Autodesk Inventor part; units mm, degrees
(part 3 of 3)
sketch "スケッチ5" plane through (0, 0, 6) normal (0, 0, 1) x (1, 0, 0)
  line L0 (155.6611, 116.5538) -> (164.0413, 130.0744) projected
  line L1 (164.0413, 130.0744) -> (164.3416, 130.559) projected
  arc A0 (164.3416, 130.559) -> (164.502, 130.8893) centre (161.9481, 131.9254) ccw projected
  arc A1 (164.502, 130.8893) -> (164.8829, 132.1201) centre (157.4972, 133.7312) ccw projected
  arc A2 (164.8829, 132.1201) -> (165.1789, 134.6281) centre (152.1823, 134.8905) ccw projected
  arc A3 (165.1789, 134.6281) -> (163.8683, 135.3286) centre (148.5, 105.0002) ccw projected
  arc A4 (163.8683, 135.3286) -> (161.9475, 133.6891) centre (171.3071, 124.6681) ccw projected
  arc A5 (161.9475, 133.6891) -> (161.1357, 132.6886) centre (167.3903, 128.4432) ccw projected
  arc A6 (161.1357, 132.6886) -> (160.9502, 132.3718) centre (163.4161, 131.1408) ccw projected
  line L2 (160.9502, 132.3718) -> (160.7141, 131.8528) projected
  arc A7 (160.7141, 131.8528) -> (158.8509, 132.6246) centre (148.5, 105.0002) ccw projected
  line L3 (158.8509, 132.6246) -> (159.051, 133.1584) projected
  arc A8 (159.051, 133.1584) -> (159.1439, 133.5137) centre (156.4368, 134.0317) ccw projected
  arc A9 (159.1439, 133.5137) -> (159.2773, 134.7951) centre (151.7192, 134.9344) ccw projected
  arc A10 (159.2773, 134.7951) -> (159.0783, 137.3127) centre (146.2802, 135.0346) ccw projected
  arc A11 (159.0783, 137.3127) -> (157.6563, 137.744) centre (148.5, 105.0002) ccw projected
  arc A12 (157.6563, 137.744) -> (156.0922, 135.7613) centre (167.0319, 128.7396) ccw projected
  arc A13 (156.0922, 135.7613) -> (155.4912, 134.6217) centre (162.4539, 131.678) ccw projected
  arc A14 (155.4912, 134.6217) -> (155.371, 134.2747) centre (158.0297, 133.5485) ccw projected
  line L4 (155.371, 134.2747) -> (155.2407, 133.7197) projected
  arc A15 (155.2407, 133.7197) -> (153.2628, 134.1131) centre (148.5, 105.0002) ccw projected
  line L5 (153.2628, 134.1131) -> (153.3548, 134.6758) projected
  arc A16 (153.3548, 134.6758) -> (153.3766, 135.0423) centre (150.6206, 135.0222) ccw projected
  arc A17 (153.3766, 135.0423) -> (153.2575, 136.3252) centre (145.8174, 134.9872) ccw projected
  arc A18 (153.2575, 136.3252) -> (152.5712, 138.7555) centre (140.4634, 134.0244) ccw projected
  arc A19 (152.5712, 138.7555) -> (151.0923, 138.9012) centre (148.5, 105.0002) ccw projected
  arc A20 (151.0923, 138.9012) -> (149.9451, 136.6514) centre (162.0444, 131.8989) ccw projected
  arc A21 (149.9451, 136.6514) -> (149.5779, 135.4165) centre (156.9811, 133.8877) ccw projected
  arc A22 (149.5779, 135.4165) -> (149.5278, 135.0527) centre (152.2771, 134.8591) ccw projected
  line L6 (149.5278, 135.0527) -> (149.5083, 134.4829) projected
  arc A23 (149.5083, 134.4829) -> (147.4916, 134.4829) centre (148.5, 105.0002) ccw projected
  line L7 (147.4916, 134.4829) -> (147.4721, 135.0527) projected
  arc A24 (147.4721, 135.0527) -> (147.422, 135.4165) centre (144.7228, 134.8591) ccw projected
  arc A25 (147.422, 135.4165) -> (147.0549, 136.6514) centre (140.0188, 133.8877) ccw projected
  arc A26 (147.0549, 136.6514) -> (145.9076, 138.9012) centre (134.9555, 131.8989) ccw projected
  arc A27 (145.9076, 138.9012) -> (144.4287, 138.7555) centre (148.5, 105.0002) ccw projected
  arc A28 (144.4287, 138.7555) -> (143.7424, 136.3252) centre (156.5365, 134.0244) ccw projected
  arc A29 (143.7424, 136.3252) -> (143.6233, 135.0423) centre (151.1825, 134.9872) ccw projected
  arc A30 (143.6233, 135.0423) -> (143.6451, 134.6758) centre (146.3794, 135.0222) ccw projected
  line L8 (143.6451, 134.6758) -> (143.7371, 134.1131) projected
  arc A31 (143.7371, 134.1131) -> (141.7592, 133.7197) centre (148.5, 105.0002) ccw projected
  line L9 (141.7592, 133.7197) -> (141.6289, 134.2747) projected
  arc A32 (141.6289, 134.2747) -> (141.5088, 134.6217) centre (138.9702, 133.5485) ccw projected
  arc A33 (141.5088, 134.6217) -> (140.9078, 135.7613) centre (134.5461, 131.678) ccw projected
  arc A34 (140.9078, 135.7613) -> (139.3437, 137.744) centre (129.9681, 128.7396) ccw projected
  arc A35 (139.3437, 137.744) -> (137.9216, 137.3127) centre (148.5, 105.0002) ccw projected
  arc A36 (137.9216, 137.3127) -> (137.7227, 134.7951) centre (150.7197, 135.0346) ccw projected
  arc A37 (137.7227, 134.7951) -> (137.8561, 133.5137) centre (145.2808, 134.9344) ccw projected
  arc A38 (137.8561, 133.5137) -> (137.949, 133.1584) centre (140.5631, 134.0317) ccw projected
  line L10 (137.949, 133.1584) -> (138.149, 132.6246) projected
  arc A39 (138.149, 132.6246) -> (136.2858, 131.8528) centre (148.5, 105.0002) ccw projected
  line L11 (136.2858, 131.8528) -> (136.0497, 132.3718) projected
  arc A40 (136.0497, 132.3718) -> (135.8642, 132.6886) centre (133.5838, 131.1408) ccw projected
  arc A41 (135.8642, 132.6886) -> (135.0525, 133.6891) centre (129.6096, 128.4432) ccw projected
  arc A42 (135.0525, 133.6891) -> (133.1316, 135.3286) centre (125.6928, 124.6681) ccw projected
  arc A43 (133.1316, 135.3286) -> (131.821, 134.6281) centre (148.5, 105.0002) ccw projected
  arc A44 (131.821, 134.6281) -> (132.117, 132.1201) centre (144.8176, 134.8905) ccw projected
  arc A45 (132.117, 132.1201) -> (132.4979, 130.8893) centre (139.5027, 133.7312) ccw projected
  arc A46 (132.4979, 130.8893) -> (132.6583, 130.559) centre (135.0518, 131.9254) ccw projected
  line L12 (132.6583, 130.559) -> (132.9586, 130.0744) projected
  arc A47 (132.9586, 130.0744) -> (131.2818, 128.954) centre (148.5, 105.0002) ccw projected
  line L13 (131.2818, 128.954) -> (130.949, 129.4169) projected
  arc A48 (130.949, 129.4169) -> (130.7053, 129.6915) centre (128.7706, 127.7285) ccw projected
  arc A49 (130.7053, 129.6915) -> (129.7139, 130.5144) centre (125.3991, 124.3074) ccw projected
  arc A50 (129.7139, 130.5144) -> (127.5101, 131.7476) centre (122.294, 119.8407) ccw projected
  arc A51 (127.5101, 131.7476) -> (126.3614, 130.8049) centre (148.5, 105.0002) ccw projected
  arc A52 (126.3614, 130.8049) -> (127.141, 128.4028) centre (139.0571, 133.5978) ccw projected
  arc A53 (127.141, 128.4028) -> (127.7546, 127.27) centre (134.0705, 131.4238) ccw projected
  arc A54 (127.7546, 127.27) -> (127.9764, 126.9773) centre (130.0574, 128.7845) ccw projected
  line L14 (127.9764, 126.9773) -> (128.3655, 126.5606) projected
  arc A55 (128.3655, 126.5606) -> (126.9395, 125.1346) centre (148.5, 105.0002) ccw projected
  line L15 (126.9395, 125.1346) -> (126.5228, 125.5237) projected
  arc A56 (126.5228, 125.5237) -> (126.2301, 125.7455) centre (124.7157, 123.4427) ccw projected
  arc A57 (126.2301, 125.7455) -> (125.0973, 126.3591) centre (122.0763, 119.4296) ccw projected
  arc A58 (125.0973, 126.3591) -> (122.6952, 127.1387) centre (119.9023, 114.4431) ccw projected
  arc A59 (122.6952, 127.1387) -> (121.7525, 125.99) centre (148.5, 105.0002) ccw projected
  arc A60 (121.7525, 125.99) -> (122.9858, 123.7862) centre (133.6594, 131.2061) ccw projected
  arc A61 (122.9858, 123.7862) -> (123.8086, 122.7949) centre (129.1927, 128.1011) ccw projected
  arc A62 (123.8086, 122.7949) -> (124.0832, 122.5511) centre (125.7717, 124.7295) ccw projected
  line L16 (124.0832, 122.5511) -> (124.5462, 122.2183) projected
  arc A63 (124.5462, 122.2183) -> (123.4257, 120.5415) centre (148.5, 105.0002) ccw projected
  line L17 (123.4257, 120.5415) -> (122.9411, 120.8418) projected
  arc A64 (122.9411, 120.8418) -> (122.6108, 121.0022) centre (121.5747, 118.4483) ccw projected
  arc A65 (122.6108, 121.0022) -> (121.3801, 121.3831) centre (119.769, 113.9974) ccw projected
  arc A66 (121.3801, 121.3831) -> (118.8721, 121.6791) centre (118.6096, 108.6825) ccw projected
  arc A67 (118.8721, 121.6791) -> (118.1715, 120.3685) centre (148.5, 105.0002) ccw projected
  arc A68 (118.1715, 120.3685) -> (119.811, 118.4477) centre (128.832, 127.8073) ccw projected
  arc A69 (119.811, 118.4477) -> (120.8115, 117.6359) centre (125.057, 123.8905) ccw projected
  arc A70 (120.8115, 117.6359) -> (121.1284, 117.4504) centre (122.3594, 119.9163) ccw projected
  line L18 (121.1284, 117.4504) -> (121.6473, 117.2143) projected
  arc A71 (121.6473, 117.2143) -> (120.8756, 115.3511) centre (148.5, 105.0002) ccw projected
  line L19 (120.8756, 115.3511) -> (120.3417, 115.5512) projected
  arc A72 (120.3417, 115.5512) -> (119.9864, 115.644) centre (119.4685, 112.937) ccw projected
  arc A73 (119.9864, 115.644) -> (118.705, 115.7775) centre (118.5657, 108.2194) ccw projected
  arc A74 (118.705, 115.7775) -> (116.1874, 115.5785) centre (118.4655, 102.7804) ccw projected
  arc A75 (116.1874, 115.5785) -> (115.7561, 114.1565) centre (148.5, 105.0002) ccw projected
  arc A76 (115.7561, 114.1565) -> (117.7388, 112.5923) centre (124.7605, 123.5321) ccw projected
  arc A77 (117.7388, 112.5923) -> (118.8784, 111.9914) centre (121.8221, 118.9541) ccw projected
  arc A78 (118.8784, 111.9914) -> (119.2254, 111.8712) centre (119.9517, 114.5299) ccw projected
  line L20 (119.2254, 111.8712) -> (119.7804, 111.7409) projected
  arc A79 (119.7804, 111.7409) -> (119.387, 109.763) centre (148.5, 105.0002) ccw projected
  line L21 (119.387, 109.763) -> (118.8243, 109.855) projected
  arc A80 (118.8243, 109.855) -> (118.4578, 109.8768) centre (118.4779, 107.1208) ccw projected
  arc A81 (118.4578, 109.8768) -> (117.175, 109.7577) centre (118.5129, 102.3176) ccw projected
  arc A82 (117.175, 109.7577) -> (114.7446, 109.0714) centre (119.4757, 96.9636) ccw projected
  arc A83 (114.7446, 109.0714) -> (114.5989, 107.5925) centre (148.5, 105.0002) ccw projected
  arc A84 (114.5989, 107.5925) -> (116.8487, 106.4453) centre (121.6012, 118.5446) ccw projected
  arc A85 (116.8487, 106.4453) -> (118.0837, 106.0781) centre (119.6124, 113.4813) ccw projected
  arc A86 (118.0837, 106.0781) -> (118.4474, 106.028) centre (118.641, 108.7773) ccw projected
  line L22 (118.4474, 106.028) -> (119.0172, 106.0085) projected
  arc A87 (119.0172, 106.0085) -> (119.0172, 103.9918) centre (148.5, 105.0002) ccw projected
  line L23 (119.0172, 103.9918) -> (118.4474, 103.9723) projected
  arc A88 (118.4474, 103.9723) -> (118.0837, 103.9222) centre (118.641, 101.223) ccw projected
  arc A89 (118.0837, 103.9222) -> (116.8487, 103.5551) centre (119.6124, 96.519) ccw projected
  arc A90 (116.8487, 103.5551) -> (114.5989, 102.4078) centre (121.6012, 91.4557) ccw projected
  arc A91 (114.5989, 102.4078) -> (114.7446, 100.9289) centre (148.5, 105.0002) ccw projected
  arc A92 (114.7446, 100.9289) -> (117.175, 100.2426) centre (119.4757, 113.0367) ccw projected
  arc A93 (117.175, 100.2426) -> (118.4578, 100.1235) centre (118.5129, 107.6827) ccw projected
  arc A94 (118.4578, 100.1235) -> (118.8243, 100.1453) centre (118.4779, 102.8796) ccw projected
  line L24 (118.8243, 100.1453) -> (119.387, 100.2373) projected
  arc A95 (119.387, 100.2373) -> (119.7804, 98.2594) centre (148.5, 105.0002) ccw projected
  line L25 (119.7804, 98.2594) -> (119.2254, 98.1291) projected
  arc A96 (119.2254, 98.1291) -> (118.8784, 98.009) centre (119.9517, 95.4704) ccw projected
  arc A97 (118.8784, 98.009) -> (117.7388, 97.408) centre (121.8221, 91.0463) ccw projected
  arc A98 (117.7388, 97.408) -> (115.7561, 95.8439) centre (124.7605, 86.4683) ccw projected
  arc A99 (115.7561, 95.8439) -> (116.1874, 94.4218) centre (148.5, 105.0002) ccw projected
  arc A100 (116.1874, 94.4218) -> (118.705, 94.2229) centre (118.4655, 107.2199) ccw projected
  arc A101 (118.705, 94.2229) -> (119.9864, 94.3563) centre (118.5657, 101.781) ccw projected
  arc A102 (119.9864, 94.3563) -> (120.3417, 94.4491) centre (119.4685, 97.0633) ccw projected
  line L26 (120.3417, 94.4491) -> (120.8756, 94.6492) projected
  arc A103 (120.8756, 94.6492) -> (121.6473, 92.786) centre (148.5, 105.0002) ccw projected
  line L27 (121.6473, 92.786) -> (121.1284, 92.5499) projected
  arc A104 (121.1284, 92.5499) -> (120.8115, 92.3644) centre (122.3594, 90.084) ccw projected
  arc A105 (120.8115, 92.3644) -> (119.811, 91.5526) centre (125.057, 86.1098) ccw projected
  arc A106 (119.811, 91.5526) -> (118.1715, 89.6318) centre (128.832, 82.193) ccw projected
  arc A107 (118.1715, 89.6318) -> (118.8721, 88.3212) centre (148.5, 105.0002) ccw projected
  arc A108 (118.8721, 88.3212) -> (121.3801, 88.6172) centre (118.6096, 101.3178) ccw projected
  arc A109 (121.3801, 88.6172) -> (122.6108, 88.9981) centre (119.769, 96.0029) ccw projected
  arc A110 (122.6108, 88.9981) -> (122.9411, 89.1585) centre (121.5747, 91.552) ccw projected
  line L28 (122.9411, 89.1585) -> (123.4257, 89.4588) projected
  arc A111 (123.4257, 89.4588) -> (124.5462, 87.782) centre (148.5, 105.0002) ccw projected
  line L29 (124.5462, 87.782) -> (124.0832, 87.4492) projected
  arc A112 (124.0832, 87.4492) -> (123.8086, 87.2055) centre (125.7717, 85.2708) ccw projected
  arc A113 (123.8086, 87.2055) -> (122.9858, 86.2141) centre (129.1927, 81.8993) ccw projected
  arc A114 (122.9858, 86.2141) -> (121.7525, 84.0103) centre (133.6594, 78.7942) ccw projected
  arc A115 (121.7525, 84.0103) -> (122.6952, 82.8616) centre (148.5, 105.0002) ccw projected
  arc A116 (122.6952, 82.8616) -> (125.0973, 83.6412) centre (119.9023, 95.5573) ccw projected
  arc A117 (125.0973, 83.6412) -> (126.2301, 84.2548) centre (122.0763, 90.5707) ccw projected
  arc A118 (126.2301, 84.2548) -> (126.5228, 84.4766) centre (124.7157, 86.5576) ccw projected
  line L30 (126.5228, 84.4766) -> (126.9395, 84.8657) projected
  arc A119 (126.9395, 84.8657) -> (128.3655, 83.4397) centre (148.5, 105.0002) ccw projected
  line L31 (128.3655, 83.4397) -> (127.9764, 83.023) projected
  arc A120 (127.9764, 83.023) -> (127.7546, 82.7303) centre (130.0574, 81.2159) ccw projected
  arc A121 (127.7546, 82.7303) -> (127.141, 81.5975) centre (134.0705, 78.5765) ccw projected
  arc A122 (127.141, 81.5975) -> (126.3614, 79.1954) centre (139.0571, 76.4025) ccw projected
  arc A123 (126.3614, 79.1954) -> (127.5101, 78.2527) centre (148.5, 105.0002) ccw projected
  arc A124 (127.5101, 78.2527) -> (129.7139, 79.486) centre (122.294, 90.1596) ccw projected
  arc A125 (129.7139, 79.486) -> (130.7053, 80.3088) centre (125.3991, 85.6929) ccw projected
  arc A126 (130.7053, 80.3088) -> (130.949, 80.5834) centre (128.7706, 82.2718) ccw projected
  line L32 (130.949, 80.5834) -> (131.2818, 81.0464) projected
  arc A127 (131.2818, 81.0464) -> (132.9586, 79.9259) centre (148.5, 105.0002) ccw projected
  line L33 (132.9586, 79.9259) -> (132.6583, 79.4413) projected
  arc A128 (132.6583, 79.4413) -> (132.4979, 79.111) centre (135.0518, 78.0749) ccw projected
  arc A129 (132.4979, 79.111) -> (132.117, 77.8803) centre (139.5027, 76.2692) ccw projected
  arc A130 (132.117, 77.8803) -> (131.821, 75.3722) centre (144.8176, 75.1098) ccw projected
  arc A131 (131.821, 75.3722) -> (133.1316, 74.6717) centre (148.5, 105.0002) ccw projected
  arc A132 (133.1316, 74.6717) -> (135.0525, 76.3112) centre (125.6928, 85.3322) ccw projected
  arc A133 (135.0525, 76.3112) -> (135.8642, 77.3117) centre (129.6096, 81.5572) ccw projected
  arc A134 (135.8642, 77.3117) -> (136.0497, 77.6286) centre (133.5838, 78.8596) ccw projected
  line L34 (136.0497, 77.6286) -> (136.2858, 78.1475) projected
  arc A135 (136.2858, 78.1475) -> (138.149, 77.3758) centre (148.5, 105.0002) ccw projected
  line L35 (138.149, 77.3758) -> (137.949, 76.8419) projected
  arc A136 (137.949, 76.8419) -> (137.8561, 76.4866) centre (140.5631, 75.9687) ccw projected
  arc A137 (137.8561, 76.4866) -> (137.7227, 75.2052) centre (145.2808, 75.0659) ccw projected
  arc A138 (137.7227, 75.2052) -> (137.9216, 72.6876) centre (150.7197, 74.9657) ccw projected
  arc A139 (137.9216, 72.6876) -> (139.3437, 72.2563) centre (148.5, 105.0002) ccw projected
  arc A140 (139.3437, 72.2563) -> (140.9078, 74.239) centre (129.9681, 81.2607) ccw projected
  arc A141 (140.9078, 74.239) -> (141.5088, 75.3786) centre (134.5461, 78.3223) ccw projected
  arc A142 (141.5088, 75.3786) -> (141.6289, 75.7256) centre (138.9702, 76.4519) ccw projected
  line L36 (141.6289, 75.7256) -> (141.7592, 76.2806) projected
  line L37 (141.7592, 76.2806) -> (145.5995, 92.6427) projected
  arc A143 (150.4672, 96.5002) -> (145.5995, 92.6427) centre (150.4672, 91.5002) ccw projected
  line L38 (150.4672, 96.5002) -> (198.5, 96.5002) projected
  line L39 (198.5, 96.5002) -> (198.5, 97.2542) projected
  arc A144 (200, 99.1907) -> (198.5, 97.2542) centre (200.5, 97.2542) ccw projected
  arc A145 (200, 99.1907) -> (202.7811, 100.7964) centre (198.5, 105.0002) ccw projected
  arc A146 (205.2082, 101.1272) -> (202.7811, 100.7964) centre (204.2082, 99.3951) ccw projected
  line L40 (205.2082, 101.1272) -> (205.8612, 100.7502) projected
  arc A147 (205.8612, 100.7502) -> (205.8612, 109.2502) centre (198.5, 105.0002) ccw projected
  line L41 (205.8612, 109.2502) -> (205.2082, 108.8731) projected
  arc A148 (202.7811, 109.2039) -> (205.2082, 108.8731) centre (204.2082, 110.6052) ccw projected
  arc A149 (202.7811, 109.2039) -> (200, 110.8096) centre (198.5, 105.0002) ccw projected
  arc A150 (198.5, 112.7461) -> (200, 110.8096) centre (200.5, 112.7461) ccw projected
  line L42 (198.5, 112.7461) -> (198.5, 113.5002) projected
  line L43 (198.5, 113.5002) -> (157.361, 113.5002) projected
  arc A151 (155.6611, 116.5538) -> (157.361, 113.5002) centre (157.361, 115.5002) ccw projected
  circle A152 centre (148.5, 105.0002) radius 2.995 projected
  circle A153 centre (201.6754, 105.0002) radius 1.5 projected
  circle A154 centre (196.9122, 107.7502) radius 1.5 projected
  circle A155 centre (196.9122, 102.2502) radius 1.5 projected
  arc A156 (161.4072, 125.8245) -> (142.9017, 81.1483) centre (148.5, 105.0002) ccw
  circle A157 centre (148.5, 105.0002) radius 7.995
  line L44 (158.1568, 130.0713) -> (146.261, 110.8786)
  line L45 (137.7989, 81.2895) -> (142.4351, 101.0422)
  line L46 (155.6611, 116.5538) -> (164.0413, 130.0744) projected
  line L47 (141.7592, 76.2806) -> (145.5995, 92.6427) projected
  line L48 (148.5, 105.0002) -> (124.8304, 114.8044) construction
  line L49 (149.4567, 107.3099) -> (125.7871, 117.1141)
  line L50 (123.8737, 112.4947) -> (147.5433, 102.6905)
  arc A158 (147.5433, 102.6905) -> (149.4567, 107.3099) centre (148.5, 105.0002) ccw
  arc A159 (125.7871, 117.1141) -> (123.8737, 112.4947) centre (124.8304, 114.8044) ccw
  circle A160 centre (196.9122, 107.7502) radius 4.5
  circle A161 centre (196.9122, 102.2502) radius 4.5
  line L51 (193.3503, 110.5002) -> (150.8097, 110.5002)
  line L52 (193.3503, 99.5002) -> (150.8097, 99.5002)
  line L53 (193.3503, 99.5002) -> (180.3344, 110.5002) construction
  line L54 (194.3185, 100.6458) -> (181.3026, 111.6458)
  line L55 (179.3662, 109.3545) -> (192.3821, 98.3545)
  arc A162 (192.3821, 98.3545) -> (194.3185, 100.6458) centre (193.3503, 99.5002) ccw
  arc A163 (181.3026, 111.6458) -> (179.3662, 109.3545) centre (180.3344, 110.5002) ccw
  line L56 (180.3344, 110.5002) -> (167.3185, 99.5002) construction
  line L57 (179.3662, 111.6458) -> (166.3502, 100.6458)
  line L58 (168.2867, 98.3545) -> (181.3026, 109.3545)
  arc A164 (181.3026, 109.3545) -> (179.3662, 111.6458) centre (180.3344, 110.5002) ccw
  arc A165 (166.3502, 100.6458) -> (168.2867, 98.3545) centre (167.3185, 99.5002) ccw
  line L59 (167.3185, 99.5002) -> (154.3025, 110.5002) construction
  line L60 (168.2867, 100.6458) -> (155.2708, 111.6458)
  line L61 (153.3343, 109.3545) -> (166.3502, 98.3545)
  arc A166 (166.3502, 98.3545) -> (168.2867, 100.6458) centre (167.3185, 99.5002) ccw
  arc A167 (155.2708, 111.6458) -> (153.3343, 109.3545) centre (154.3025, 110.5002) ccw
  point P0 (0, 0)
  point P1 (136.6652, 109.9023)
  point P2 (186.8423, 105.0002)
  point P3 (173.8264, 105.0002)
  point P4 (160.8105, 105.0002)
  point P5 (182.6582, 110.5002)
  point P6 (192.4123, 102.2568)
  point P7 (193.3503, 105.0002)
  point P8 (180.3344, 108.5362)
  point P9 (169.6423, 99.5002)
  point P10 (191.0265, 99.5002)
  point P11 (164.9946, 99.5002)
  point P12 (156.273, 106.871)
  point P13 (154.3025, 99.5002)
  point P14 (156.6264, 110.5002)
  point P15 (167.3185, 101.4641)
  point P16 (178.0105, 110.5002)
  point P17 (140.5272, 105.5966)
  point P18 (125.0264, 112.0173)
  point P19 (138.1518, 82.7928)
  point P20 (142.2067, 100.0691)
  point P21 (126.9398, 116.6367)
  point P22 (142.4407, 110.216)
  point P23 (147.5367, 112.9369)
  point P24 (156.8856, 128.0204)
  dimension "d28" = 5
  dimension "d29" = 5
  dimension "d30" = 5
  dimension "d31" = 5
  dimension "d32" = 5
  dimension "d33" = 99.291
  dimension "d34" = 99.291
  dimension "d35" = 3
  dimension "d36" = 3
  dimension "d37" = 3
  dimension "d38" = 3
  dimension "d39" = 3
  dimension "d40" = 3
  dimension "d41" = 3
  constraints: 40 end point, 18 point on circle, 16 tangent, 9 centre point, 7 parallel, 5 point on line, 4 midpoint, 2 horizontal, 1 coincident, 1 equal length, 9 other
  measures "d28" radial gap between concentric circles of A31 A156
  measures "d30" distance between parallel lines of L0 L44
  measures "d31" distance between parallel lines of L37 L45
  measures "d32" diameter of A159
  measures "d33" angle of L48 L0
  measures "d34" angle of L37 L48
  measures "d35" diameter of A154
  measures "d36" diameter of A155
  measures "d37" distance between parallel lines of L51 L43
  measures "d38" distance between parallel lines of L38 L52
  measures "d39" diameter of A163
  measures "d40" diameter of A165
  measures "d41" diameter of A167
extrude "押し出し5" cut sketch "スケッチ5" against normal blind 6 contours L44 A157 L49 A156 | L50 A157 L45 A156 | A160 A161 L54 L51 | L61 L52 A157 | L51 L57 L60 | L52 L58 L55
fillet "フィレット4" radius 1 17 edges at (156.6264, 110.5002, 3) (156.273, 106.871, 3) (154.3025, 99.5002, 3) (164.9946, 99.5002, 3) (167.3185, 101.4641, 3) (178.0105, 110.5002, 3) (180.3344, 108.5362, 3) (169.6423, 99.5002, 3) (191.0265, 99.5002, 3) (192.4123, 102.2568, 3) (193.3503, 105.0002, 3) (193.3503, 110.5002, 3) (182.6582, 110.5002, 3) (156.8856, 128.0204, 3) (126.9398, 116.6367, 3) (125.0264, 112.0173, 3) (138.1518, 82.7928, 3)
fillet "フィレット5" radius 5 4 edges at (147.5367, 112.9369, 3) (142.4407, 110.216, 3) (140.5272, 105.5966, 3) (142.2067, 100.0691, 3)
equation "\"d34\" = d33"
